Autodesk Fusion 360 part; units mm, degrees
(part 3 of 4)
combine "negative for the plate" operation cut target body 2 tool bodies 1 keep tools
extrude "remove excess" cut sketch "plate" against normal up to surface (5.4 mm away) contours A0 A1 L0 A3 A5 A6 L1 L2 L3 A7 A8 L5 L6 L7 A9 L10 L11 A11 L13 L14 A12 L18 L19 L20 L22 A13 A14 A15 A16 L23 L24 A18 L26 L27 A19 L28 L31 L32 A21 A24 A25 A29 A31 L45 A35 L46 L49 A38 L52 A39 L55 A46 A47 A106 A107 L362 A108 A109 L371 L372 A111 A114 L378 A116 L379 L381 A120 L386 A121 A122 A123 A124 L389 A125 L390 L392 L393 L397 | A10 | L77 A67 L100 A68 A69 L109 L110 L112 L114 L115 A70 L126 L128 A71 L133 A72 L145 L146 A73 L149 A74 A75 A76 L150 A77 A78 A79 L151 L152 A80 A81 L153 L154 A82 L155 L156 A83 L157 A84 L160 L161 A85 A86 L162 L163 A87 A88 A89 A90 L166 A91 A92 L167 L168 L169 A93 L170 A94 L173 A95 A96 L175 A97 L176 A98 L178 A99 L183 A100 L188 A101 A102 L197 A103 L212 A104 A105 L251 | L164 L192 L231 L241 | L209 L242 L286 L298 | L361 L370 L388 L394 | A110 | A112 | A113 | A115 | A117 | A118 | A119 | L401 A126 L402 A127 L403 A128 L404 A129 L405 A130 L406 A131 L407 A132 L408 A133 L409 A134 L410 A135 L411 A136 L412 A137 L413 A138 L414 A139 L415 A140 L416 A141 L417 A142 L418 A143 L419 A144 L420 A145 L421 A146 L422 A147 L423 A148 L424 A149 L425 A150 L426 A151 L427 A152 L428 A153 L429 A154 L430 A155 L431 A156 L432 A157 L433 A158 L434 A159 L435 A160 L436 A161 L437 A162 L438 A163 L439 A164 bodies 2
sketch "plate mounting holes" plane through (0, 0, 0) normal (0, 0, -1) x (1, 0, 0)
  arc A0 (359.744, -10) -> (352.994, -3.25) centre (352.994, -10) ccw
  line L0 (352.994, -3.25) -> (287.1404, -3.25)
  arc A1 (286.1404, -2.25) -> (287.1404, -3.25) centre (287.1404, -2.25) ccw
  line L1 (286.1404, -2.25) -> (286.1404, -1.7)
  arc A2 (286.1404, -1.7) -> (281.6404, 2.8) centre (281.6404, -1.7) ccw
  line L2 (281.6404, 2.8) -> (281.1404, 2.8)
  arc A3 (281.1404, 2.8) -> (276.6404, -1.7) centre (281.1404, -1.7) ccw
  line L3 (276.6404, -1.7) -> (276.6404, -2.25)
  arc A4 (275.6404, -3.25) -> (276.6404, -2.25) centre (275.6404, -2.25) ccw
  line L4 (275.6404, -3.25) -> (209.7869, -3.25)
  arc A5 (208.8748, -3.1702) -> (209.7869, -3.25) centre (209.7869, 2) ccw
  line L5 (208.8748, -3.1702) -> (184.7261, 1.0897)
  arc A6 (183.915, 2.2482) -> (184.7261, 1.0897) centre (184.8998, 2.0745) ccw
  line L6 (183.915, 2.2482) -> (184.0105, 2.7899)
  arc A7 (184.0105, 2.7899) -> (180.3607, 8.0032) centre (179.579, 3.5716) ccw
  line L7 (180.3607, 8.0032) -> (179.8683, 8.09)
  arc A8 (179.8683, 8.09) -> (174.655, 4.4402) centre (179.0866, 3.6585) ccw
  line L8 (174.655, 4.4402) -> (174.5594, 3.8986)
  arc A9 (173.4009, 3.0875) -> (174.5594, 3.8986) centre (173.5747, 4.0723) ccw
  line L9 (173.4009, 3.0875) -> (149.2522, 7.3474)
  arc A10 (149.2522, 7.3474) -> (146.212, 7.3474) centre (147.7321, -1.2696) ccw
  line L10 (146.212, 7.3474) -> (122.0657, 3.0876)
  arc A11 (120.9071, 3.8986) -> (122.0657, 3.0876) centre (121.8919, 4.0724) ccw
  line L11 (120.9071, 3.8986) -> (120.8116, 4.4403)
  arc A12 (120.8116, 4.4403) -> (115.5982, 8.09) centre (116.38, 3.6585) ccw
  line L12 (115.5982, 8.09) -> (115.1058, 8.0032)
  arc A13 (115.1058, 8.0032) -> (111.4561, 2.7898) centre (115.8876, 3.5716) ccw
  line L13 (111.4561, 2.7898) -> (111.5516, 2.2482)
  arc A14 (110.7406, 1.0896) -> (111.5516, 2.2482) centre (110.5668, 2.0744) ccw
  line L14 (110.7406, 1.0896) -> (86.5943, -3.1702)
  arc A15 (85.6822, -3.25) -> (86.5943, -3.1702) centre (85.6822, 2) ccw
  line L15 (85.6822, -3.25) -> (49.5915, -3.25)
  arc A16 (48.5915, -2.25) -> (49.5915, -3.25) centre (49.5915, -2.25) ccw
  line L16 (48.5915, -2.25) -> (48.5915, -1.7)
  arc A17 (48.5915, -1.7) -> (44.0915, 2.8) centre (44.0915, -1.7) ccw
  line L17 (44.0915, 2.8) -> (43.5915, 2.8)
  arc A18 (43.5915, 2.8) -> (39.0915, -1.7) centre (43.5915, -1.7) ccw
  line L18 (39.0915, -1.7) -> (39.0915, -2.25)
  arc A19 (38.0915, -3.25) -> (39.0915, -2.25) centre (38.0915, -2.25) ccw
  line L19 (38.0915, -3.25) -> (2.0009, -3.25)
  arc A20 (2.0009, -3.25) -> (-4.7491, -10) centre (2.0009, -10) ccw
  line L20 (-4.7491, -10) -> (-4.7491, -110.024)
  arc A21 (-4.7491, -110.024) -> (2.0009, -116.774) centre (2.0009, -110.024) ccw
  line L21 (2.0009, -116.774) -> (40.125, -116.774)
  arc A22 (41.125, -117.774) -> (40.125, -116.774) centre (40.125, -117.774) ccw
  line L22 (41.125, -117.774) -> (41.125, -118.324)
  arc A23 (41.125, -118.324) -> (45.625, -122.824) centre (45.625, -118.324) ccw
  line L23 (45.625, -122.824) -> (46.125, -122.824)
  arc A24 (46.125, -122.824) -> (50.625, -118.324) centre (46.125, -118.324) ccw
  line L24 (50.625, -118.324) -> (50.625, -117.774)
  arc A25 (51.625, -116.774) -> (50.625, -117.774) centre (51.625, -117.774) ccw
  line L25 (51.625, -116.774) -> (127.8733, -116.774)
  arc A26 (128.8733, -117.774) -> (127.8733, -116.774) centre (127.8733, -117.774) ccw
  line L26 (128.8733, -117.774) -> (128.8733, -118.324)
  arc A27 (128.8733, -118.324) -> (133.3733, -122.824) centre (133.3733, -118.324) ccw
  line L27 (133.3733, -122.824) -> (133.8733, -122.824)
  arc A28 (133.8733, -122.824) -> (138.3733, -118.324) centre (133.8733, -118.324) ccw
  line L28 (138.3733, -118.324) -> (138.3733, -117.774)
  arc A29 (139.3733, -116.774) -> (138.3733, -117.774) centre (139.3733, -117.774) ccw
  line L29 (139.3733, -116.774) -> (215.6216, -116.774)
  arc A30 (216.6216, -117.774) -> (215.6216, -116.774) centre (215.6216, -117.774) ccw
  line L30 (216.6216, -117.774) -> (216.6216, -118.324)
  arc A31 (216.6216, -118.324) -> (221.1216, -122.824) centre (221.1216, -118.324) ccw
  line L31 (221.1216, -122.824) -> (221.6216, -122.824)
  arc A32 (221.6216, -122.824) -> (226.1216, -118.324) centre (221.6216, -118.324) ccw
  line L32 (226.1216, -118.324) -> (226.1216, -117.774)
  arc A33 (227.1216, -116.774) -> (226.1216, -117.774) centre (227.1216, -117.774) ccw
  line L33 (227.1216, -116.774) -> (303.3699, -116.774)
  arc A34 (304.3699, -117.774) -> (303.3699, -116.774) centre (303.3699, -117.774) ccw
  line L34 (304.3699, -117.774) -> (304.3699, -118.324)
  arc A35 (304.3699, -118.324) -> (308.8699, -122.824) centre (308.8699, -118.324) ccw
  line L35 (308.8699, -122.824) -> (309.3699, -122.824)
  arc A36 (309.3699, -122.824) -> (313.8699, -118.324) centre (309.3699, -118.324) ccw
  line L36 (313.8699, -118.324) -> (313.8699, -117.774)
  arc A37 (314.8699, -116.774) -> (313.8699, -117.774) centre (314.8699, -117.774) ccw
  line L37 (314.8699, -116.774) -> (352.994, -116.774)
  arc A38 (352.994, -116.774) -> (359.744, -110.024) centre (352.994, -110.024) ccw
  line L38 (359.744, -110.024) -> (359.744, -10)
  line L39 (42.375, -118.324) -> (42.375, -117.774)
  arc A39 (42.375, -117.774) -> (40.125, -115.524) centre (40.125, -117.774) ccw
  line L40 (40.125, -115.524) -> (2.0009, -115.524)
  arc A40 (-3.4991, -110.024) -> (2.0009, -115.524) centre (2.0009, -110.024) ccw
  line L41 (-3.4991, -110.024) -> (-3.4991, -10)
  arc A41 (2.0009, -4.5) -> (-3.4991, -10) centre (2.0009, -10) ccw
  line L42 (2.0009, -4.5) -> (38.0915, -4.5)
  arc A42 (38.0915, -4.5) -> (40.3415, -2.25) centre (38.0915, -2.25) ccw
  line L43 (40.3415, -2.25) -> (40.3415, -1.7)
  arc A43 (43.5915, 1.55) -> (40.3415, -1.7) centre (43.5915, -1.7) ccw
  line L44 (43.5915, 1.55) -> (44.0915, 1.55)
  arc A44 (47.3415, -1.7) -> (44.0915, 1.55) centre (44.0915, -1.7) ccw
  line L45 (47.3415, -1.7) -> (47.3415, -2.25)
  arc A45 (47.3415, -2.25) -> (49.5915, -4.5) centre (49.5915, -2.25) ccw
  line L46 (49.5915, -4.5) -> (85.6822, -4.5)
  arc A46 (85.6822, -4.5) -> (86.8114, -4.4012) centre (85.6822, 2) ccw
  line L47 (86.8114, -4.4012) -> (110.9577, -0.1414)
  arc A47 (110.9577, -0.1414) -> (112.7826, 2.4653) centre (110.5668, 2.0744) ccw
  line L48 (112.7826, 2.4653) -> (112.687, 3.007)
  arc A48 (115.323, 6.7722) -> (112.687, 3.007) centre (115.8876, 3.5716) ccw
  line L49 (115.323, 6.7722) -> (115.8154, 6.859)
  arc A49 (119.5806, 4.2231) -> (115.8154, 6.859) centre (116.38, 3.6585) ccw
  line L50 (119.5806, 4.2231) -> (119.6762, 3.6815)
  arc A50 (119.6762, 3.6815) -> (122.2828, 1.8566) centre (121.8919, 4.0724) ccw
  line L51 (122.2828, 1.8566) -> (146.4291, 6.1164)
  arc A51 (149.035, 6.1164) -> (146.4291, 6.1164) centre (147.7321, -1.2696) ccw
  line L52 (149.035, 6.1164) -> (173.1838, 1.8565)
  arc A52 (173.1838, 1.8565) -> (175.7904, 3.6814) centre (173.5747, 4.0723) ccw
  line L53 (175.7904, 3.6814) -> (175.886, 4.2231)
  arc A53 (179.6512, 6.859) -> (175.886, 4.2231) centre (179.0866, 3.6585) ccw
  line L54 (179.6512, 6.859) -> (180.1436, 6.7722)
  arc A54 (182.7796, 3.007) -> (180.1436, 6.7722) centre (179.579, 3.5716) ccw
  line L55 (182.7796, 3.007) -> (182.684, 2.4654)
  arc A55 (182.684, 2.4654) -> (184.5089, -0.1413) centre (184.8998, 2.0745) ccw
  line L56 (184.5089, -0.1413) -> (208.6577, -4.4012)
  arc A56 (208.6577, -4.4012) -> (209.7869, -4.5) centre (209.7869, 2) ccw
  line L57 (209.7869, -4.5) -> (275.6404, -4.5)
  arc A57 (275.6404, -4.5) -> (277.8904, -2.25) centre (275.6404, -2.25) ccw
  line L58 (277.8904, -2.25) -> (277.8904, -1.7)
  arc A58 (281.1404, 1.55) -> (277.8904, -1.7) centre (281.1404, -1.7) ccw
  line L59 (281.1404, 1.55) -> (281.6404, 1.55)
  arc A59 (284.8904, -1.7) -> (281.6404, 1.55) centre (281.6404, -1.7) ccw
  line L60 (284.8904, -1.7) -> (284.8904, -2.25)
  arc A60 (284.8904, -2.25) -> (287.1404, -4.5) centre (287.1404, -2.25) ccw
  line L61 (287.1404, -4.5) -> (352.994, -4.5)
  arc A61 (358.494, -10) -> (352.994, -4.5) centre (352.994, -10) ccw
  line L62 (358.494, -10) -> (358.494, -110.024)
  arc A62 (352.994, -115.524) -> (358.494, -110.024) centre (352.994, -110.024) ccw
  line L63 (352.994, -115.524) -> (314.8699, -115.524)
  arc A63 (314.8699, -115.524) -> (312.6199, -117.774) centre (314.8699, -117.774) ccw
  line L64 (312.6199, -117.774) -> (312.6199, -118.324)
  arc A64 (309.3699, -121.574) -> (312.6199, -118.324) centre (309.3699, -118.324) ccw
  line L65 (309.3699, -121.574) -> (308.8699, -121.574)
  arc A65 (305.6199, -118.324) -> (308.8699, -121.574) centre (308.8699, -118.324) ccw
  line L66 (305.6199, -118.324) -> (305.6199, -117.774)
  arc A66 (305.6199, -117.774) -> (303.3699, -115.524) centre (303.3699, -117.774) ccw
  line L67 (303.3699, -115.524) -> (227.1216, -115.524)
  arc A67 (227.1216, -115.524) -> (224.8716, -117.774) centre (227.1216, -117.774) ccw
  line L68 (224.8716, -117.774) -> (224.8716, -118.324)
  arc A68 (221.6216, -121.574) -> (224.8716, -118.324) centre (221.6216, -118.324) ccw
  line L69 (221.6216, -121.574) -> (221.1216, -121.574)
  arc A69 (217.8716, -118.324) -> (221.1216, -121.574) centre (221.1216, -118.324) ccw
  line L70 (217.8716, -118.324) -> (217.8716, -117.774)
  arc A70 (217.8716, -117.774) -> (215.6216, -115.524) centre (215.6216, -117.774) ccw
  line L71 (215.6216, -115.524) -> (139.3733, -115.524)
  arc A71 (139.3733, -115.524) -> (137.1233, -117.774) centre (139.3733, -117.774) ccw
  line L72 (137.1233, -117.774) -> (137.1233, -118.324)
  arc A72 (133.8733, -121.574) -> (137.1233, -118.324) centre (133.8733, -118.324) ccw
  line L73 (133.8733, -121.574) -> (133.3733, -121.574)
  arc A73 (130.1233, -118.324) -> (133.3733, -121.574) centre (133.3733, -118.324) ccw
  line L74 (130.1233, -118.324) -> (130.1233, -117.774)
  arc A74 (130.1233, -117.774) -> (127.8733, -115.524) centre (127.8733, -117.774) ccw
  line L75 (127.8733, -115.524) -> (51.625, -115.524)
  arc A75 (51.625, -115.524) -> (49.375, -117.774) centre (51.625, -117.774) ccw
  line L76 (49.375, -117.774) -> (49.375, -118.324)
  arc A76 (46.125, -121.574) -> (49.375, -118.324) centre (46.125, -118.324) ccw
  line L77 (46.125, -121.574) -> (45.625, -121.574)
  arc A77 (42.375, -118.324) -> (45.625, -121.574) centre (45.625, -118.324) ccw
  circle A78 centre (309.1199, -118.074) radius 1.55 construction
  circle A79 centre (221.3716, -118.074) radius 1.55 construction
  circle A80 centre (133.6233, -118.074) radius 1.55 construction
  circle A81 centre (45.875, -118.074) radius 1.55 construction
  circle A82 centre (43.8415, -1.95) radius 1.55 construction
  circle A83 centre (116.1773, 3.3688) radius 1.55 construction
  circle A84 centre (179.2893, 3.3688) radius 1.55 construction
  circle A85 centre (281.3904, -1.95) radius 1.55 construction
  circle A86 centre (43.8415, -1.95) radius 1.5
  circle A87 centre (116.1773, 3.3688) radius 1.5
  circle A88 centre (179.2893, 3.3688) radius 1.5
  circle A89 centre (281.3904, -1.95) radius 1.5
  circle A90 centre (309.1199, -118.074) radius 1.5
  circle A91 centre (221.3716, -118.074) radius 1.5
  circle A92 centre (133.6233, -118.074) radius 1.5
  circle A93 centre (45.875, -118.074) radius 1.5
  dimension "d59" = 3
  dimension "d60" = 3
  dimension "d61" = 3
  dimension "d62" = 3
  dimension "d63" = 3
  dimension "d64" = 3
  dimension "d65" = 3
  dimension "d66" = 3
  constraint concentric A82 A86
  constraint concentric A83 A87
  constraint concentric A84 A88
  constraint concentric A85 A89
  constraint concentric A78 A90
  constraint concentric A79 A91
  constraint concentric A80 A92
  constraint concentric A81 A93
  measures "d59" diameter of A86
  measures "d60" diameter of A87
  measures "d61" diameter of A88
  measures "d62" diameter of A89
  measures "d63" diameter of A90
  measures "d64" diameter of A91
  measures "d65" diameter of A92
  measures "d66" diameter of A93
extrude "top case mouning holes" cut sketch "plate mounting holes" against normal blind 2.4 contours A86 | A87 | A88 | A89 | A90 | A91 | A92 | A93 bodies 2
thread "Thread1" "ISO Metric profile 3.0 M3x0.5 6H" major diameter 3.086 minor diameter 2.529 pitch 0.5 angle 60 resizes the face on face at (310.1672, 117.0002, 1.6) on bodies 2
thread "Thread2" "ISO Metric profile 3.0 M3x0.5 6H" major diameter 3.086 minor diameter 2.529 pitch 0.5 angle 60 resizes the face on face at (221.7779, 116.6301, 1.6) on bodies 2
thread "Thread3" "ISO Metric profile 3.0 M3x0.5 6H" major diameter 3.086 minor diameter 2.529 pitch 0.5 angle 60 resizes the face on face at (134.2402, 116.7067, 1.6) on bodies 2
thread "Thread4" "ISO Metric profile 3.0 M3x0.5 6H" major diameter 3.086 minor diameter 2.529 pitch 0.5 angle 60 resizes the face on face at (47.2573, 117.4913, 1.6) on bodies 2
thread "Thread5" "ISO Metric profile 3.0 M3x0.5 6H" major diameter 3.086 minor diameter 2.529 pitch 0.5 angle 60 resizes the face on face at (44.2478, 0.5061, 1.6) on bodies 2
thread "Thread6" "ISO Metric profile 3.0 M3x0.5 6H" major diameter 3.086 minor diameter 2.529 pitch 0.5 angle 60 resizes the face on face at (116.5835, -4.8128, 1.6) on bodies 2
thread "Thread7" "ISO Metric profile 3.0 M3x0.5 6H" major diameter 3.086 minor diameter 2.529 pitch 0.5 angle 60 resizes the face on face at (179.9063, -4.7361, 1.6) on bodies 2
thread "Thread8" "ISO Metric profile 3.0 M3x0.5 6H" major diameter 3.086 minor diameter 2.529 pitch 0.5 angle 60 resizes the face on face at (280.3979, 3.0747, 1.6) on bodies 2
chamfer "Chamfer1" distance 3.5 angle 45 13 edges at (97.494, -6.1147, 6.6) (127.2167, -11.3582, 6.6) (147.732, -14.7304, 6.6) (180.2368, -9.2436, 6.6) (281.478, -4, 6.6) (362.8935, 0.1005, 6.6) (366.994, 60.012, 6.6) (362.8935, 119.9235, 6.6) (177.4975, 124.024, 6.6) (-7.8986, 119.9235, 6.6) (-11.9991, 60.012, 6.6) (-7.8986, 0.1005, 6.6) (43.754, -4, 6.6) on bodies 2
sketch "Bottom" plane through (0, 0, -5.4) normal (0, 0, -1) x (1, 0, 0)
  arc A0 (38.0915, -3.25) -> (39.0915, -2.25) centre (38.0915, -2.25) ccw
  line L0 (39.0915, -2.25) -> (39.0915, -1.7)
  arc A1 (43.5915, 2.8) -> (39.0915, -1.7) centre (43.5915, -1.7) ccw
  line L1 (43.5915, 2.8) -> (44.0915, 2.8)
  arc A2 (48.5915, -1.7) -> (44.0915, 2.8) centre (44.0915, -1.7) ccw
  line L2 (48.5915, -1.7) -> (48.5915, -2.25)
  arc A3 (48.5915, -2.25) -> (49.5915, -3.25) centre (49.5915, -2.25) ccw
  line L3 (49.5915, -3.25) -> (85.6822, -3.25)
  arc A4 (85.6822, -3.25) -> (86.5943, -3.1702) centre (85.6822, 2) ccw
  line L4 (86.5943, -3.1702) -> (110.7406, 1.0896)
  arc A5 (110.7406, 1.0896) -> (111.5516, 2.2482) centre (110.5668, 2.0744) ccw
  line L5 (111.5516, 2.2482) -> (111.4561, 2.7898)
  arc A6 (115.1058, 8.0032) -> (111.4561, 2.7898) centre (115.8876, 3.5716) ccw
  line L6 (115.1058, 8.0032) -> (115.5982, 8.09)
  arc A7 (120.8116, 4.4403) -> (115.5982, 8.09) centre (116.38, 3.6585) ccw
  line L7 (120.8116, 4.4403) -> (120.9071, 3.8986)
  arc A8 (120.9071, 3.8986) -> (122.0657, 3.0876) centre (121.8919, 4.0724) ccw
  line L8 (122.0657, 3.0876) -> (146.212, 7.3474)
  arc A9 (149.2522, 7.3474) -> (146.212, 7.3474) centre (147.7321, -1.2696) ccw
  line L9 (149.2522, 7.3474) -> (173.4009, 3.0875)
  arc A10 (173.4009, 3.0875) -> (174.5594, 3.8986) centre (173.5747, 4.0723) ccw
  line L10 (174.5594, 3.8986) -> (174.655, 4.4402)
  arc A11 (179.8683, 8.09) -> (174.655, 4.4402) centre (179.0866, 3.6585) ccw
  line L11 (179.8683, 8.09) -> (180.3607, 8.0032)
  arc A12 (184.0105, 2.7899) -> (180.3607, 8.0032) centre (179.579, 3.5716) ccw
  line L12 (184.0105, 2.7899) -> (183.915, 2.2482)
  arc A13 (183.915, 2.2482) -> (184.7261, 1.0897) centre (184.8998, 2.0745) ccw
  line L13 (184.7261, 1.0897) -> (208.8748, -3.1702)
  arc A14 (208.8748, -3.1702) -> (209.7869, -3.25) centre (209.7869, 2) ccw
  line L14 (209.7869, -3.25) -> (275.6404, -3.25)
  arc A15 (275.6404, -3.25) -> (276.6404, -2.25) centre (275.6404, -2.25) ccw
  line L15 (276.6404, -2.25) -> (276.6404, -1.7)
  arc A16 (281.1404, 2.8) -> (276.6404, -1.7) centre (281.1404, -1.7) ccw
  line L16 (281.1404, 2.8) -> (281.6404, 2.8)
  arc A17 (286.1404, -1.7) -> (281.6404, 2.8) centre (281.6404, -1.7) ccw
  line L17 (286.1404, -1.7) -> (286.1404, -2.25)
  arc A18 (286.1404, -2.25) -> (287.1404, -3.25) centre (287.1404, -2.25) ccw
  line L18 (287.1404, -3.25) -> (352.994, -3.25)
  arc A19 (359.744, -10) -> (352.994, -3.25) centre (352.994, -10) ccw
  line L19 (359.744, -10) -> (359.744, -110.024)
  arc A20 (352.994, -116.774) -> (359.744, -110.024) centre (352.994, -110.024) ccw
  line L20 (352.994, -116.774) -> (314.8699, -116.774)
  arc A21 (314.8699, -116.774) -> (313.8699, -117.774) centre (314.8699, -117.774) ccw
  line L21 (313.8699, -117.774) -> (313.8699, -118.324)
  arc A22 (309.3699, -122.824) -> (313.8699, -118.324) centre (309.3699, -118.324) ccw
  line L22 (309.3699, -122.824) -> (308.8699, -122.824)
  arc A23 (304.3699, -118.324) -> (308.8699, -122.824) centre (308.8699, -118.324) ccw
  line L23 (304.3699, -118.324) -> (304.3699, -117.774)
  arc A24 (304.3699, -117.774) -> (303.3699, -116.774) centre (303.3699, -117.774) ccw
  line L24 (303.3699, -116.774) -> (227.1216, -116.774)
  arc A25 (227.1216, -116.774) -> (226.1216, -117.774) centre (227.1216, -117.774) ccw
  line L25 (226.1216, -117.774) -> (226.1216, -118.324)
  arc A26 (221.6216, -122.824) -> (226.1216, -118.324) centre (221.6216, -118.324) ccw
  line L26 (221.6216, -122.824) -> (221.1216, -122.824)
  arc A27 (216.6216, -118.324) -> (221.1216, -122.824) centre (221.1216, -118.324) ccw
  line L27 (216.6216, -118.324) -> (216.6216, -117.774)
  arc A28 (216.6216, -117.774) -> (215.6216, -116.774) centre (215.6216, -117.774) ccw
  line L28 (215.6216, -116.774) -> (139.3733, -116.774)
  arc A29 (139.3733, -116.774) -> (138.3733, -117.774) centre (139.3733, -117.774) ccw
  line L29 (138.3733, -117.774) -> (138.3733, -118.324)
  arc A30 (133.8733, -122.824) -> (138.3733, -118.324) centre (133.8733, -118.324) ccw
  line L30 (133.8733, -122.824) -> (133.3733, -122.824)
  arc A31 (128.8733, -118.324) -> (133.3733, -122.824) centre (133.3733, -118.324) ccw
  line L31 (128.8733, -118.324) -> (128.8733, -117.774)
  arc A32 (128.8733, -117.774) -> (127.8733, -116.774) centre (127.8733, -117.774) ccw
  line L32 (127.8733, -116.774) -> (51.625, -116.774)
  arc A33 (51.625, -116.774) -> (50.625, -117.774) centre (51.625, -117.774) ccw
  line L33 (50.625, -117.774) -> (50.625, -118.324)
  arc A34 (46.125, -122.824) -> (50.625, -118.324) centre (46.125, -118.324) ccw
  line L34 (46.125, -122.824) -> (45.625, -122.824)
  arc A35 (41.125, -118.324) -> (45.625, -122.824) centre (45.625, -118.324) ccw
  line L35 (41.125, -118.324) -> (41.125, -117.774)
  arc A36 (41.125, -117.774) -> (40.125, -116.774) centre (40.125, -117.774) ccw
  line L36 (40.125, -116.774) -> (2.0009, -116.774)
  arc A37 (-4.7491, -110.024) -> (2.0009, -116.774) centre (2.0009, -110.024) ccw
  line L37 (-4.7491, -110.024) -> (-4.7491, -10)
  arc A38 (2.0009, -3.25) -> (-4.7491, -10) centre (2.0009, -10) ccw
  line L38 (2.0009, -3.25) -> (38.0915, -3.25)
  arc A39 (352.994, -124.024) -> (366.994, -110.024) centre (352.994, -110.024) ccw
  line L39 (366.994, -110.024) -> (366.994, -10)
  arc A40 (366.994, -10) -> (352.994, 4) centre (352.994, -10) ccw
  line L40 (352.994, 4) -> (209.9619, 4)
  line L41 (209.9619, 4) -> (150.5116, 14.4871)
  arc A41 (150.5116, 14.4871) -> (144.9524, 14.4871) centre (147.7321, -1.2696) ccw
  line L42 (144.9524, 14.4871) -> (109.481, 8.2294)
  line L43 (109.481, 8.2294) -> (85.5071, 4)
  line L44 (85.5071, 4) -> (2.0009, 4)
  arc A42 (2.0009, 4) -> (-11.9991, -10) centre (2.0009, -10) ccw
  line L45 (-11.9991, -10) -> (-11.9991, -110.024)
  arc A43 (-11.9991, -110.024) -> (2.0009, -124.024) centre (2.0009, -110.024) ccw
  line L46 (2.0009, -124.024) -> (352.994, -124.024)
  line L47 (2.0009, -124.024) -> (352.994, -124.024)
  arc A44 (-11.9991, -110.024) -> (2.0009, -124.024) centre (2.0009, -110.024) ccw
  line L48 (-11.9991, -10) -> (-11.9991, -110.024)
  arc A45 (2.0009, 4) -> (-11.9991, -10) centre (2.0009, -10) ccw
  line L49 (85.5071, 4) -> (2.0009, 4)
  line L50 (109.481, 8.2294) -> (85.5071, 4)
  line L51 (144.9524, 14.4871) -> (109.481, 8.2294)
  arc A46 (150.5116, 14.4871) -> (144.9524, 14.4871) centre (147.7321, -1.2696) ccw
  line L52 (209.9619, 4) -> (150.5116, 14.4871)
  line L53 (352.994, 4) -> (209.9619, 4)
  arc A47 (366.994, -10) -> (352.994, 4) centre (352.994, -10) ccw
  line L54 (366.994, -110.024) -> (366.994, -10)
  arc A48 (352.994, -124.024) -> (366.994, -110.024) centre (352.994, -110.024) ccw
extrude "bottom extrude" add sketch "Bottom" along normal blind 18 separate body contours A0 L0 A1 L1 A2 L2 A3 L3 A4 L4 A5 L5 A6 L6 A7 L7 A8 L8 A9 L9 A10 L10 A11 L11 A12 L12 A13 L13 A14 L14 A15 L15 A16 L16 A17 L17 A18 L18 A19 L19 A20 L20 A21 L21 A22 L22 A23 L23 A24 L24 A25 L25 A26 L26 A27 L27 A28 L28 A29 L29 A30 L30 A31 L31 A32 L32 A33 L33 A34 L34 A35 L35 A36 L36 A37 L37 A38 L38 | A39 L39 A40 L40 L41 A41 L42 L43 L44 A42 L45 A43 L46 L47 A44 L48 A45 L49 L50 L51 A46 L52 L53 A47 L54 A48 makes body 3
sketch "side profile" plane through (366.994, 0, 0) normal (1, 0, 0) x (0, 1, 0)
  line L0 (110.024, -5.4) -> (10, -5.4)
  line L1 (10, -5.4) -> (10, -23.4)
  line L2 (10, -23.4) -> (110.024, -23.4)
  line L3 (110.024, -23.4) -> (110.024, -5.4)
  line L4 (-14.4871, -5.4) -> (-14.4871, -23.4)
  line L5 (124.024, -21.7169) -> (-14.4871, -9.5988)
  line L6 (-14.4871, -23.4) -> (124.137, -27.0751)
  line L7 (124.024, -5.4) -> (124.024, -23.4)
  line L8 (124.024, -23.4) -> (124.137, -27.0751)
  dimension "d85" = 85
  constraint coincident L4 L5.end
  constraint coincident L4.end L6.start
  constraint coincident L5.start L7
  constraint coincident L7.end L8.start
  measures "d85" angle of L5 L7
extrude "bottom cut" cut sketch "side profile" against normal up to surface (378.9931 mm away) contours L1 L2 L3 L4 L5 L6 L7 L8 | L1 L2 L3 L5 bodies 3
delete_face "DeleteFace1" 1 faces at (148.6586, -14.4871, -14.1992) on bodies 3
shell "Shell1" thickness 7.25 removed faces 1 at (188.3189, 81.3493, -5.4) on bodies 3
ref_plane "WorkPlane3" through (177.4975, 57.0752, -3.44) normal (0, 0, -1) x (-1, 0, 0)
sketch "usb c cutout" plane through (0, 124.024, 0) normal (0, 1, 0) x (-1, 0, 0)
  line L0 (-2.0009, 3.1) -> (-352.994, 3.1)
  line L1 (-352.994, 3.1) -> (-352.994, -5.4)
  line L2 (-352.994, -5.4) -> (-2.0009, -5.4)
  line L3 (-2.0009, -5.4) -> (-2.0009, 3.1)
  line L4 (-146.7359, -4.04) -> (-146.7359, -2.04)
  arc A0 (-146.7359, -2.04) -> (-147.2359, -1.54) centre (-147.2359, -2.04) ccw
  line L5 (-147.2359, -1.54) -> (-155.1859, -1.54)
  arc A1 (-155.1859, -1.54) -> (-155.6859, -2.04) centre (-155.1859, -2.04) ccw
  line L6 (-155.6859, -2.04) -> (-155.6859, -4.04)
  arc A2 (-155.6859, -4.04) -> (-155.1859, -4.54) centre (-155.1859, -4.04) ccw
  arc A3 (-147.2359, -4.54) -> (-146.7359, -4.04) centre (-147.2359, -4.04) ccw
  line L7 (-155.1859, -4.54) -> (-147.2359, -4.54)
  line L8 (-157.3109, -2.04) -> (-157.3109, -4.04)
  arc A4 (-157.3109, -4.04) -> (-155.1859, -6.165) centre (-155.1859, -4.04) ccw
  line L9 (-155.1859, -6.165) -> (-147.2359, -6.165)
  arc A5 (-147.2359, -6.165) -> (-145.1109, -4.04) centre (-147.2359, -4.04) ccw
  line L10 (-145.1109, -4.04) -> (-145.1109, -2.04)
  arc A6 (-145.1109, -2.04) -> (-147.2359, 0.085) centre (-147.2359, -2.04) ccw
  line L11 (-147.2359, 0.085) -> (-155.1859, 0.085)
  arc A7 (-155.1859, 0.085) -> (-157.3109, -2.04) centre (-155.1859, -2.04) ccw
  dimension "d97" = 1.625
extrude "Extrude10" cut sketch "usb c cutout" against normal up to surface (8.5 mm away) contours L2 A4 L9 A5 | L2 L8 A4 A5 L10 A6 L11 A7 | L4 A0 L5 A1 L6 A2 A3 L7 bodies 2 3
chamfer "Chamfer2" distance 0.75 angle 45 10 edges at (157.1841, 124.024, -4.7632) (157.3109, 124.024, -3.04) (156.6885, 124.024, -0.5374) (151.2109, 124.024, 0.085) (145.7333, 124.024, -0.5374) (145.1109, 124.024, -3.04) (145.2377, 124.024, -4.7632) (146.3343, 124.024, -5.9643) (151.2109, 124.024, -6.165) (156.0875, 124.024, -5.9643) on bodies 2 3
ref_plane "WorkPlane4" through (177.4975, 60.012, 0.6) normal (1, 0, 0) x (0, 1, 0)
sketch "encoder inlay" plane through (0, 0, 6.6) normal (0, 0, 1) x (-1, 0, 0)
  circle A0 centre (-342.9945, -61.9242) radius 4.125
  circle A1 centre (-333.4695, -100.0241) radius 4.125
  circle A2 centre (-338.232, -80.9741) radius 4.125
  line L0 (-85.8135, 0.5) -> (-110.0891, 4.7826)
  line L1 (-110.0891, 4.7826) -> (-145.5605, 11.0403)
  arc A3 (-145.5605, 11.0403) -> (-149.9036, 11.0404) centre (-147.7321, -1.2696) ccw
  line L2 (-149.9036, 11.0404) -> (-209.6556, 0.5)
  line L3 (-209.6556, 0.5) -> (-352.994, 0.5)
  arc A4 (-352.994, 0.5) -> (-363.494, -10) centre (-352.994, -10) ccw
  line L4 (-363.494, -10) -> (-363.494, -110.024)
  arc A5 (-363.494, -110.024) -> (-352.994, -120.524) centre (-352.994, -110.024) ccw
  line L5 (-352.994, -120.524) -> (-2.0009, -120.524)
  arc A6 (-2.0009, -120.524) -> (8.4991, -110.024) centre (-2.0009, -110.024) ccw
  line L6 (8.4991, -110.024) -> (8.4991, -10)
  arc A7 (8.4991, -10) -> (-2.0009, 0.5) centre (-2.0009, -10) ccw
  line L7 (-2.0009, 0.5) -> (-85.8135, 0.5)
  circle A8 centre (-333.4695, -100.0241) radius 7.5
  circle A9 centre (-338.232, -80.9741) radius 7.5
  circle A10 centre (-342.9945, -61.9242) radius 7.5
  arc A11 (-64.4423, -14.5796) -> (-65.7943, -12.6489) centre (-66.0837, -14.2903) ccw
  line L8 (-64.4423, -14.5796) -> (-67.1459, -29.9138)
  arc A12 (-67.1459, -29.9138) -> (-65.6759, -31.861) centre (-65.5045, -30.2032) ccw
  arc A13 (-65.6759, -31.861) -> (-49.9524, -32.8112) centre (-46.6903, 151.7378) ccw
  arc A14 (-49.9524, -32.8112) -> (-48.2563, -31.1489) centre (-49.923, -31.1448) ccw
  line L9 (-48.2563, -31.1489) -> (-48.218, -15.452)
  arc A15 (-46.5508, -13.7894) -> (-48.218, -15.452) centre (-46.5514, -15.4561) ccw
  line L10 (-46.5508, -13.7894) -> (-1.2271, -13.8044)
  arc A16 (0.439, -15.4793) -> (-1.2271, -13.8044) centre (-1.2277, -15.471) ccw
  line L11 (0.439, -15.4793) -> (0.2609, -51.2421)
  arc A17 (-1.3993, -52.9005) -> (0.2609, -51.2421) centre (-1.4058, -51.2338) ccw
  line L12 (-1.3993, -52.9005) -> (-2.4426, -52.9046)
  line L13 (-2.4426, -52.9046) -> (-2.4294, -70.2787)
  arc A18 (-4.0987, -71.9466) -> (-2.4294, -70.2787) centre (-4.0961, -70.28) ccw
  line L14 (-4.0987, -71.9466) -> (-4.3438, -71.9462)
  line L15 (-4.3438, -71.9462) -> (-4.3309, -89.333)
  arc A19 (-5.9963, -91.0009) -> (-4.3309, -89.333) centre (-5.9976, -89.3342) ccw
  line L16 (-5.9963, -91.0009) -> (-9.1197, -91.0032)
  line L17 (-9.1197, -91.0032) -> (-9.1197, -108.4579)
  arc A20 (-10.7898, -110.1245) -> (-9.1197, -108.4579) centre (-10.7864, -108.4579) ccw
  line L18 (-10.7898, -110.1245) -> (-47.2272, -110.05)
  arc A21 (-47.2272, -110.05) -> (-47.9484, -110.2125) centre (-47.2306, -111.7167) ccw
  line L19 (-47.9484, -110.2125) -> (-52.543, -112.405)
  arc A22 (-53.553, -112.5417) -> (-52.543, -112.405) centre (-53.2608, -110.9008) ccw
  line L20 (-53.553, -112.5417) -> (-145.7402, -96.1274)
  arc A23 (-147.0899, -94.1998) -> (-145.7402, -96.1274) centre (-145.448, -94.4865) ccw
  line L21 (-147.0899, -94.1998) -> (-144.2409, -77.8876)
  arc A24 (-142.3095, -76.533) -> (-144.2409, -77.8876) centre (-142.5991, -78.1743) ccw
  line L22 (-142.3095, -76.533) -> (-134.7109, -77.8736)
  line L23 (-134.7109, -77.8736) -> (-131.5483, -60.1855)
  line L24 (-131.5483, -60.1855) -> (-134.562, -59.6601)
  arc A25 (-135.9169, -57.7279) -> (-134.562, -59.6601) centre (-134.2757, -58.0182) ccw
  line L25 (-135.9169, -57.7279) -> (-132.8787, -40.5527)
  line L26 (-132.8787, -40.5527) -> (-140.6605, -39.1866)
  arc A26 (-142.0131, -37.2523) -> (-140.6605, -39.1866) centre (-140.3723, -37.5451) ccw
  line L27 (-142.0131, -37.2523) -> (-138.9556, -20.1149)
  line L28 (-138.9556, -20.1149) -> (-141.7354, -19.6252)
  arc A27 (-143.0876, -17.6947) -> (-141.7354, -19.6252) centre (-141.4462, -17.9838) ccw
  line L29 (-143.0876, -17.6947) -> (-140.1864, -1.2256)
  arc A28 (-138.2556, 0.1266) -> (-140.1864, -1.2256) centre (-138.545, -1.5147) ccw
  line L30 (-138.2556, 0.1266) -> (-65.7943, -12.6489)
  arc A29 (-290.104, -10.7013) -> (-291.7706, -9.0321) centre (-291.7707, -10.6987) ccw
  line L31 (-290.104, -10.7013) -> (-290.1298, -27.3847)
  arc A30 (-291.7971, -29.0488) -> (-290.1298, -27.3847) centre (-291.7965, -27.3821) ccw
  line L32 (-291.7971, -29.0488) -> (-309.1522, -29.0421)
  line L33 (-309.1522, -29.0421) -> (-309.1294, -46.3914)
  arc A31 (-310.7973, -48.0603) -> (-309.1294, -46.3914) centre (-310.796, -46.3936) ccw
  line L34 (-310.7973, -48.0603) -> (-327.619, -48.0472)
  arc A32 (-329.2843, -46.3744) -> (-327.619, -48.0472) centre (-327.6177, -46.3805) ccw
  line L35 (-329.2843, -46.3744) -> (-329.2213, -29.0938)
  line L36 (-329.2213, -29.0938) -> (-346.5912, -29.0945)
  arc A33 (-348.2579, -27.4277) -> (-346.5912, -29.0945) centre (-346.5913, -27.4278) ccw
  line L37 (-348.2579, -27.4277) -> (-348.2569, -10.6952)
  arc A34 (-346.5901, -9.0287) -> (-348.2569, -10.6952) centre (-346.5902, -10.6953) ccw
  line L38 (-346.5901, -9.0287) -> (-291.7706, -9.0321)
  arc A35 (-164.5843, -2.8728) -> (-166.5156, -1.521) centre (-166.2256, -3.1623) ccw
  line L39 (-164.5843, -2.8728) -> (-161.566, -19.9855)
  line L40 (-161.566, -19.9855) -> (-158.3407, -19.4167)
  arc A36 (-156.4098, -20.7686) -> (-158.3407, -19.4167) centre (-158.0512, -21.058) ccw
  line L41 (-156.4098, -20.7686) -> (-153.5181, -37.1669)
  arc A37 (-154.8721, -39.098) -> (-153.5181, -37.1669) centre (-155.1595, -37.4563) ccw
  line L42 (-154.8721, -39.098) -> (-162.6093, -40.4525)
  line L43 (-162.6093, -40.4525) -> (-159.4763, -58.2214)
  line L44 (-159.4763, -58.2214) -> (-156.4246, -57.6876)
  arc A38 (-154.4961, -59.04) -> (-156.4246, -57.6876) centre (-156.1374, -59.3294) ccw
  line L45 (-154.4961, -59.04) -> (-151.5886, -75.5295)
  arc A39 (-152.9422, -77.4605) -> (-151.5886, -75.5295) centre (-153.23, -75.8189) ccw
  line L46 (-152.9422, -77.4605) -> (-160.6851, -78.8178)
  line L47 (-160.6851, -78.8178) -> (-157.6604, -96.0106)
  arc A40 (-159.0128, -97.9408) -> (-157.6604, -96.0106) centre (-159.3018, -96.2994) ccw
  line L48 (-159.0128, -97.9408) -> (-232.6973, -110.9171)
  arc A41 (-233.2721, -110.9177) -> (-232.6973, -110.9171) centre (-232.9864, -109.2757) ccw
  line L49 (-233.2721, -110.9177) -> (-238.1216, -110.0736)
  arc A42 (-238.1216, -110.0736) -> (-238.407, -110.049) centre (-238.4074, -111.7156) ccw
  line L50 (-238.407, -110.049) -> (-313.2527, -110.0326)
  arc A43 (-314.919, -108.3659) -> (-313.2527, -110.0326) centre (-313.2523, -108.3659) ccw
  line L51 (-314.919, -108.3659) -> (-314.919, -91.0499)
  line L52 (-314.919, -91.0499) -> (-318.0141, -91.0512)
  arc A44 (-319.6815, -89.3845) -> (-318.0141, -91.0512) centre (-318.0148, -89.3845) ccw
  line L53 (-319.6815, -89.3845) -> (-319.6815, -72.0042)
  line L54 (-319.6815, -72.0042) -> (-319.919, -72.0043)
  arc A45 (-321.5862, -70.3377) -> (-319.919, -72.0043) centre (-319.9196, -70.3377) ccw
  line L55 (-321.5862, -70.3377) -> (-321.5862, -53.627)
  arc A46 (-319.9205, -51.9603) -> (-321.5862, -53.627) centre (-319.9196, -53.627) ccw
  line L56 (-319.9205, -51.9603) -> (-305.3937, -51.9521)
  line L57 (-305.3937, -51.9521) -> (-305.3937, -34.5947)
  arc A47 (-303.7283, -32.928) -> (-305.3937, -34.5947) centre (-303.7271, -34.5947) ccw
  line L58 (-303.7283, -32.928) -> (-286.3442, -32.9149)
  line L59 (-286.3442, -32.9149) -> (-286.3442, -15.4662)
  arc A48 (-284.6776, -13.7995) -> (-286.3442, -15.4662) centre (-284.6776, -15.4662) ccw
  line L60 (-284.6776, -13.7995) -> (-239.3858, -13.7995)
  arc A49 (-237.7191, -15.4662) -> (-239.3858, -13.7995) centre (-239.3858, -15.4662) ccw
  line L61 (-237.7191, -15.4662) -> (-237.7191, -31.0628)
  arc A50 (-237.7191, -31.0628) -> (-235.9174, -32.724) centre (-236.0525, -31.0628) ccw
  arc A51 (-235.9174, -32.724) -> (-229.6794, -31.998) centre (-243.2466, 57.4136) ccw
  arc A52 (-229.6794, -31.998) -> (-228.2881, -30.061) centre (-229.9295, -30.3502) ccw
  line L62 (-228.2881, -30.061) -> (-231.0106, -14.6069)
  arc A53 (-229.6592, -12.6764) -> (-231.0106, -14.6069) centre (-229.3692, -14.3177) ccw
  line L63 (-229.6592, -12.6764) -> (-166.5156, -1.521)
  dimension "d103" = 15
  dimension "d104" = 15
  dimension "d105" = 15
  constraint concentric A1 A8
  constraint concentric A2 A9
  constraint concentric A0 A10
  measures "d103" diameter of A8
  measures "d104" diameter of A9
  measures "d105" diameter of A10
extrude "encoder inlay (1)" cut sketch "encoder inlay" against normal blind 4.6 contours A8 | A9 | A10 bodies 2
chamfer "encoder chamfer" distance 0.5 angle 45 6 edges at (349.987, 59.212, 6.6) (346.8404, 63.4158, 2) (345.2245, 78.262, 6.6) (342.0779, 82.4658, 2) (337.3154, 101.5158, 2) (340.462, 97.312, 6.6) on bodies 2
sketch "connecting holes" plane through (0, 0, -5.4) normal (0, 0, -1) x (1, 0, 0)
  spline S0 degree 2 poles (145.6031, -123.274) (145.2205, -123.568) (144.7029, -124.024) knots 0.526349 0.526349 0.526349 0.590297 0.590297 0.590297 weights 1.215208 1.120677 1
  line L0 (145.6031, -123.274) -> (145.6031, -116.774)
  line L1 (145.6031, -116.774) -> (139.3733, -116.774)
  arc A0 (139.3733, -116.774) -> (138.3733, -117.774) centre (139.3733, -117.774) ccw
  line L2 (138.3733, -117.774) -> (138.3733, -118.324)
  arc A1 (133.8733, -122.824) -> (138.3733, -118.324) centre (133.8733, -118.324) ccw
  line L3 (133.8733, -122.824) -> (133.3733, -122.824)
  arc A2 (128.8733, -118.324) -> (133.3733, -122.824) centre (133.3733, -118.324) ccw
  line L4 (128.8733, -118.324) -> (128.8733, -117.774)
  arc A3 (128.8733, -117.774) -> (127.8733, -116.774) centre (127.8733, -117.774) ccw
  line L5 (127.8733, -116.774) -> (51.625, -116.774)
  arc A4 (51.625, -116.774) -> (50.625, -117.774) centre (51.625, -117.774) ccw
  line L6 (50.625, -117.774) -> (50.625, -118.324)
  arc A5 (46.125, -122.824) -> (50.625, -118.324) centre (46.125, -118.324) ccw
  line L7 (46.125, -122.824) -> (45.625, -122.824)
  arc A6 (41.125, -118.324) -> (45.625, -122.824) centre (45.625, -118.324) ccw
  line L8 (41.125, -118.324) -> (41.125, -117.774)
  arc A7 (41.125, -117.774) -> (40.125, -116.774) centre (40.125, -117.774) ccw
  line L9 (40.125, -116.774) -> (2.0009, -116.774)
  arc A8 (-4.7491, -110.024) -> (2.0009, -116.774) centre (2.0009, -110.024) ccw
  line L10 (-4.7491, -110.024) -> (-4.7491, -10)
  arc A9 (2.0009, -3.25) -> (-4.7491, -10) centre (2.0009, -10) ccw
  line L11 (2.0009, -3.25) -> (38.0915, -3.25)
  arc A10 (38.0915, -3.25) -> (39.0915, -2.25) centre (38.0915, -2.25) ccw
  line L12 (39.0915, -2.25) -> (39.0915, -1.7)
  arc A11 (43.5915, 2.8) -> (39.0915, -1.7) centre (43.5915, -1.7) ccw
  line L13 (43.5915, 2.8) -> (44.0915, 2.8)
  arc A12 (48.5915, -1.7) -> (44.0915, 2.8) centre (44.0915, -1.7) ccw
  line L14 (48.5915, -1.7) -> (48.5915, -2.25)
  arc A13 (48.5915, -2.25) -> (49.5915, -3.25) centre (49.5915, -2.25) ccw
  line L15 (49.5915, -3.25) -> (85.6822, -3.25)
  arc A14 (85.6822, -3.25) -> (86.5943, -3.1702) centre (85.6822, 2) ccw
  line L16 (86.5943, -3.1702) -> (110.7406, 1.0896)
  arc A15 (110.7406, 1.0896) -> (111.5516, 2.2482) centre (110.5668, 2.0744) ccw
  line L17 (111.5516, 2.2482) -> (111.4561, 2.7898)
  arc A16 (115.1058, 8.0032) -> (111.4561, 2.7898) centre (115.8876, 3.5716) ccw
  line L18 (115.1058, 8.0032) -> (115.5982, 8.09)
  arc A17 (120.8116, 4.4403) -> (115.5982, 8.09) centre (116.38, 3.6585) ccw
  line L19 (120.8116, 4.4403) -> (120.9071, 3.8986)
  arc A18 (120.9071, 3.8986) -> (122.0657, 3.0876) centre (121.8919, 4.0724) ccw
  line L20 (122.0657, 3.0876) -> (146.212, 7.3474)
  arc A19 (149.2522, 7.3474) -> (146.212, 7.3474) centre (147.7321, -1.2696) ccw
  line L21 (149.2522, 7.3474) -> (173.4009, 3.0875)
  arc A20 (173.4009, 3.0875) -> (174.5594, 3.8986) centre (173.5747, 4.0723) ccw
  line L22 (174.5594, 3.8986) -> (174.655, 4.4402)
  arc A21 (179.8683, 8.09) -> (174.655, 4.4402) centre (179.0866, 3.6585) ccw
  line L23 (179.8683, 8.09) -> (180.3607, 8.0032)
  arc A22 (184.0105, 2.7899) -> (180.3607, 8.0032) centre (179.579, 3.5716) ccw
  line L24 (184.0105, 2.7899) -> (183.915, 2.2482)
  arc A23 (183.915, 2.2482) -> (184.7261, 1.0897) centre (184.8998, 2.0745) ccw
  line L25 (184.7261, 1.0897) -> (208.8748, -3.1702)
  arc A24 (208.8748, -3.1702) -> (209.7869, -3.25) centre (209.7869, 2) ccw
  line L26 (209.7869, -3.25) -> (275.6404, -3.25)
  arc A25 (275.6404, -3.25) -> (276.6404, -2.25) centre (275.6404, -2.25) ccw
  line L27 (276.6404, -2.25) -> (276.6404, -1.7)
  arc A26 (281.1404, 2.8) -> (276.6404, -1.7) centre (281.1404, -1.7) ccw
  line L28 (281.1404, 2.8) -> (281.6404, 2.8)
  arc A27 (286.1404, -1.7) -> (281.6404, 2.8) centre (281.6404, -1.7) ccw
  line L29 (286.1404, -1.7) -> (286.1404, -2.25)
  arc A28 (286.1404, -2.25) -> (287.1404, -3.25) centre (287.1404, -2.25) ccw
  line L30 (287.1404, -3.25) -> (352.994, -3.25)
  arc A29 (359.744, -10) -> (352.994, -3.25) centre (352.994, -10) ccw
  line L31 (359.744, -10) -> (359.744, -110.024)
  arc A30 (352.994, -116.774) -> (359.744, -110.024) centre (352.994, -110.024) ccw
  line L32 (352.994, -116.774) -> (314.8699, -116.774)
  arc A31 (314.8699, -116.774) -> (313.8699, -117.774) centre (314.8699, -117.774) ccw
  line L33 (313.8699, -117.774) -> (313.8699, -118.324)
  arc A32 (309.3699, -122.824) -> (313.8699, -118.324) centre (309.3699, -118.324) ccw
  line L34 (309.3699, -122.824) -> (308.8699, -122.824)
  arc A33 (304.3699, -118.324) -> (308.8699, -122.824) centre (308.8699, -118.324) ccw
  line L35 (304.3699, -118.324) -> (304.3699, -117.774)
  arc A34 (304.3699, -117.774) -> (303.3699, -116.774) centre (303.3699, -117.774) ccw
  line L36 (303.3699, -116.774) -> (227.1216, -116.774)
  arc A35 (227.1216, -116.774) -> (226.1216, -117.774) centre (227.1216, -117.774) ccw
  line L37 (226.1216, -117.774) -> (226.1216, -118.324)
  arc A36 (221.6216, -122.824) -> (226.1216, -118.324) centre (221.6216, -118.324) ccw
  line L38 (221.6216, -122.824) -> (221.1216, -122.824)
  arc A37 (216.6216, -118.324) -> (221.1216, -122.824) centre (221.1216, -118.324) ccw
  line L39 (216.6216, -118.324) -> (216.6216, -117.774)
  arc A38 (216.6216, -117.774) -> (215.6216, -116.774) centre (215.6216, -117.774) ccw
  line L40 (215.6216, -116.774) -> (156.8187, -116.774)
  line L41 (156.8187, -116.774) -> (156.8187, -123.274)
  spline S1 degree 2 poles (157.7189, -124.024) (157.2013, -123.568) (156.8187, -123.274) knots 0 0 0 0.063947 0.063947 0.063947 weights 1 1.120677 1.215208
  line L42 (157.7189, -124.024) -> (352.994, -124.024)
  arc A39 (352.994, -124.024) -> (366.994, -110.024) centre (352.994, -110.024) ccw
  line L43 (366.994, -110.024) -> (366.994, -10)
  arc A40 (366.994, -10) -> (352.994, 4) centre (352.994, -10) ccw
  line L44 (352.994, 4) -> (209.9619, 4)
  line L45 (209.9619, 4) -> (150.5116, 14.4871)
  arc A41 (150.5116, 14.4871) -> (144.9524, 14.4871) centre (147.7321, -1.2696) ccw
  line L46 (144.9524, 14.4871) -> (109.481, 8.2294)
  line L47 (109.481, 8.2294) -> (85.5071, 4)
  line L48 (85.5071, 4) -> (2.0009, 4)
  arc A42 (2.0009, 4) -> (-11.9991, -10) centre (2.0009, -10) ccw
  line L49 (-11.9991, -10) -> (-11.9991, -110.024)
  arc A43 (-11.9991, -110.024) -> (2.0009, -124.024) centre (2.0009, -110.024) ccw
  line L50 (2.0009, -124.024) -> (144.7029, -124.024)
  arc A44 (352.994, -124.024) -> (366.994, -110.024) centre (352.994, -110.024) ccw
  arc A45 (366.994, -10) -> (352.994, 4) centre (352.994, -10) ccw
  arc A46 (150.5116, 14.4871) -> (144.9524, 14.4871) centre (147.7321, -1.2696) ccw
  arc A47 (2.0009, 4) -> (-11.9991, -10) centre (2.0009, -10) ccw
  arc A48 (-11.9991, -110.024) -> (2.0009, -124.024) centre (2.0009, -110.024) ccw
  line L51 (-11.9991, -110.024) -> (-11.9991, -10)
  line L52 (2.0009, 4) -> (85.5071, 4)
  line L53 (85.5071, 4) -> (144.9524, 14.4871)
  line L54 (150.5116, 14.4871) -> (209.9619, 4)
  line L55 (209.9619, 4) -> (352.994, 4)
  line L56 (366.994, -10) -> (366.994, -110.024)
  line L57 (352.994, -124.024) -> (2.0009, -124.024)
  arc A49 (-7.9991, -110.024) -> (2.0009, -120.024) centre (2.0009, -110.024) ccw construction
  line L58 (352.994, -120.024) -> (2.0009, -120.024) construction
  arc A50 (352.994, -120.024) -> (362.994, -110.024) centre (352.994, -110.024) ccw construction
  line L59 (362.994, -10) -> (362.994, -110.024) construction
  arc A51 (362.994, -10) -> (352.994, 0) centre (352.994, -10) ccw construction
  line L60 (209.6118, 0) -> (352.994, 0) construction
  line L61 (149.8168, 10.548) -> (209.6118, 0) construction
  arc A52 (149.8168, 10.548) -> (145.6473, 10.5479) centre (147.7321, -1.2696) ccw construction
  line L62 (85.8572, 0) -> (145.6473, 10.5479) construction
  line L63 (2.0009, 0) -> (85.8572, 0) construction
  arc A53 (2.0009, 0) -> (-7.9991, -10) centre (2.0009, -10) ccw construction
  line L64 (-7.9991, -110.024) -> (-7.9991, -10) construction
  circle A54 centre (360.0651, -117.0951) radius 1.5
  circle A55 centre (360.0651, -2.9289) radius 1.5
  circle A56 centre (-5.0702, -2.9289) radius 1.5
  circle A57 centre (-5.0702, -117.0951) radius 1.5
  circle A58 centre (85.8572, 0) radius 1.5
  circle A59 centre (209.6118, 0) radius 1.5
  circle A60 centre (147.7321, 10.7304) radius 1.5
  line L65 (85.8572, 0) -> (85.8572, -120.024) construction
  line L66 (209.6118, 0) -> (209.6118, -120.024) construction
  circle A61 centre (85.8572, -120.024) radius 1.5
  circle A62 centre (209.6118, -120.024) radius 1.5
  circle A63 centre (209.6118, -120.024) radius 2
  circle A64 centre (85.8572, -120.024) radius 1.75
  circle A65 centre (-5.0702, -117.0951) radius 1.75
  circle A66 centre (-5.0702, -2.9289) radius 1.75
  circle A67 centre (85.8572, 0) radius 1.75
  circle A68 centre (147.7321, 10.7304) radius 1.75
  circle A69 centre (209.6118, 0) radius 1.75
  circle A70 centre (360.0651, -2.9289) radius 1.75
  circle A71 centre (360.0651, -117.0951) radius 1.75
  point P0 (209.9619, 4)
  point P1 (85.5071, 4)
  dimension "d131" = -4
  dimension "d132" = 3
  dimension "d133" = 3
  dimension "d134" = 3
  dimension "d135" = 3
  dimension "d136" = 3
  dimension "d137" = 3
  dimension "d138" = 3
  dimension "d140" = 3
  dimension "d141" = 3
  dimension "d144" = 0.5
  dimension "d145" = 0.25
  dimension "d146" = 0.25
  dimension "d147" = 0.25
  dimension "d148" = 0.25
  dimension "d149" = 0.25
  dimension "d150" = 0.25
  dimension "d151" = 0.25
  dimension "d152" = 0.25
  constraint coincident L49.end A43.start
  constraint coincident A42.end L49.start
  constraint coincident L48.end A42.start
  constraint coincident P1 L47.end
  constraint coincident A41.end L46.start
  constraint coincident L45.end A41.start
  constraint coincident P0 L44.end
  constraint coincident A40.end L44.start
  constraint coincident L43.end A40.start
  constraint coincident A39.end L43.start
  constraint coincident L42.end A39.start
  constraint coincident A43.end L50.start
  constraint midpoint A50 A54.centre
  constraint midpoint A51 A55.centre
  constraint midpoint A53 A56.centre
  constraint midpoint A49 A57.centre
  constraint coincident L62.start L63.end
  constraint coincident L60.start L61.end
  constraint midpoint A52 A60.centre
  constraint coincident L58 L65.end
  constraint perpendicular L58 L65
  constraint coincident L58 L66.end
  constraint perpendicular L58 L66
  constraint coincident L65.end A61.centre
  constraint coincident L66.end A62.centre
  measures "d132" diameter of A54
  measures "d133" diameter of A55
  measures "d134" diameter of A56
  measures "d135" diameter of A57
  measures "d136" diameter of A58
  measures "d137" diameter of A59
  measures "d138" diameter of A60
  measures "d140" diameter of A61
  measures "d141" diameter of A62
extrude "holes" cut sketch "connecting holes" against normal blind 3 contours A54 | A55 | A56 | A57 | A58 | A59 | A61 | A62 bodies 2
thread "Thread9" "ISO Metric profile 3.0 M3x0.5 6H" major diameter 3.086 minor diameter 2.529 pitch 0.5 angle 60 resizes the face on face at (361.4473, 116.5124, -3.4) on bodies 2
thread "Thread10" "ISO Metric profile 3.0 M3x0.5 6H" major diameter 3.086 minor diameter 2.529 pitch 0.5 angle 60 resizes the face on face at (210.2287, 118.6567, -3.4) on bodies 2
thread "Thread11" "ISO Metric profile 3.0 M3x0.5 6H" major diameter 3.086 minor diameter 2.529 pitch 0.5 angle 60 resizes the face on face at (84.4477, 119.511, -3.4) on bodies 2
thread "Thread12" "ISO Metric profile 3.0 M3x0.5 6H" major diameter 3.086 minor diameter 2.529 pitch 0.5 angle 60 resizes the face on face at (-3.6165, 116.7249, -3.4) on bodies 2
thread "Thread13" "ISO Metric profile 3.0 M3x0.5 6H" major diameter 3.086 minor diameter 2.529 pitch 0.5 angle 60 resizes the face on face at (-3.572, 3.0037, -3.4) on bodies 2
thread "Thread14" "ISO Metric profile 3.0 M3x0.5 6H" major diameter 3.086 minor diameter 2.529 pitch 0.5 angle 60 resizes the face on face at (87.3554, 0.0748, -3.4) on bodies 2
thread "Thread16" "ISO Metric profile 3.0 M3x0.5 6H" major diameter 3.086 minor diameter 2.529 pitch 0.5 angle 60 resizes the face on face at (210.2287, -1.3673, -3.4) on bodies 2
thread "Thread17" "ISO Metric profile 3.0 M3x0.5 6H" major diameter 3.086 minor diameter 2.529 pitch 0.5 angle 60 resizes the face on face at (360.3255, 1.4517, -3.4) on bodies 2
extrude "Extrude15" cut sketch "connecting holes" along normal up to surface contours A54 | A55 | A56 | A57 | A58 | A59 | A61 | A62 | A63 | A64 | A65 | A66 | A67 | A69 | A70 | A71 end surface through (366.994, 124.024, -21.7169) normal (0, -0.087156, -0.996195) offset 0 bodies 3
ref_plane "WorkPlane6" through (177.4975, 124.024, -21.7169) normal (0, 0, 1) x (-1, 0, 0)
sketch "inlay" plane through (177.4975, 124.024, -21.7169) normal (0, 0, 1) x (1, 0, 0)
  circle A0 centre (182.5676, -6.9289) radius 1.2645
  circle A1 centre (32.1143, -4) radius 1.2645
  circle A2 centre (-91.6402, -4) radius 1.2645
  circle A3 centre (-182.5676, -6.9289) radius 1.2645
  circle A4 centre (-182.5676, -121.0951) radius 1.2645
  circle A5 centre (-91.6402, -124.024) radius 1.2645
  circle A6 centre (32.1143, -124.024) radius 1.2645
  circle A7 centre (182.5676, -121.0951) radius 1.2645
  circle A8 centre (182.5676, -6.9289) radius 2.8
  circle A9 centre (32.1143, -4) radius 2.8
  circle A10 centre (-91.6402, -4) radius 2.8
  circle A11 centre (-182.5676, -6.9289) radius 2.8
  circle A12 centre (-182.5676, -121.0951) radius 2.8
  circle A13 centre (-91.6402, -124.024) radius 2.8
  circle A14 centre (32.1143, -124.024) radius 2.8
  circle A15 centre (182.5676, -121.0951) radius 2.8
  dimension "d156" = 5.6
  dimension "d157" = 5.6
  dimension "d158" = 5.6
  dimension "d159" = 5.6
  dimension "d160" = 5.6
  dimension "d161" = 5.6
  dimension "d162" = 5.6
  dimension "d163" = 5.6
  constraint concentric A0 A8
  constraint concentric A1 A9
  constraint concentric A2 A10
  constraint concentric A3 A11
  constraint concentric A4 A12
  constraint concentric A5 A13
  constraint concentric A6 A14
  constraint concentric A7 A15
  measures "d156" diameter of A8
  measures "d157" diameter of A9
  measures "d158" diameter of A10
  measures "d159" diameter of A11
  measures "d160" diameter of A12
  measures "d161" diameter of A13
  measures "d162" diameter of A14
  measures "d163" diameter of A15
extrude "Extrude16" cut sketch "inlay" along normal blind 1.5 contours A8 | A9 | A10 | A11 bodies 3
extrude "Extrude17" cut sketch "inlay" along normal blind 11.5 contours A12 | A13 | A14 | A15 bodies 3
move_body "Move4" bodies 2 3 1 to x (1, 0, 0) y (0, 0.996195, 0.087156) z (0, -0.087156, 0.996195) at (0, 0.3566, -4.9683)